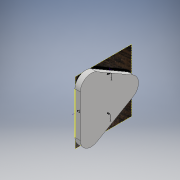
# Autodesk Inventor part: frontHub
Saved by Autodesk Inventor 2018 (Build 220112000, 112)
## iProperties
Created: 2019-07-29
Part Number: frontHub
Material: Generic
Document SubType Name: Modeling
Designer: Aditya Kendre
Density: 1 g/cm^3
Appearance: Default
Author: Aditya Kendre
Autodesk Inventor part; units mm, degrees
ref_plane "YZ Plane" through (0, 0, 0) normal (1, 0, 0) x (0, 1, 0)
ref_plane "XZ Plane" through (0, 0, 0) normal (0, 1, 0) x (-1, 0, 0)
ref_plane "XY Plane" through (0, 0, 0) normal (0, 0, 1) x (1, 0, 0)
sketch "Sketch1" plane through (0, 0, 0) normal (1, 0, 0) x (0, 1, 0)
  line L0 (0, 0) -> (12.7, 0) construction
  line L1 (12.7, 0) -> (-6.35, -10.9985)
  line L2 (-6.35, -10.9985) -> (-6.35, 10.9985)
  line L3 (-6.35, 10.9985) -> (12.7, 0)
  dimension "d0" = 12.7
  constraints: 8 end point, 1 coincident, 1 horizontal, 7 other
  measures "d0" distance of L0.start L0.end
extrude "Extrusion1" add sketch "Sketch1" along normal blind 1.5
fillet "Fillet1" radius 3 3 edges at (0.75, 12.7, 0) (0.75, -6.35, 10.9985) (0.75, -6.35, -10.9985)
sketch "Sketch2" plane through (0, 0, 0) normal (-1, 0, 0) x (0, 0, 1)
  line L0 (2.5981, 8.2) -> (8.4004, -1.85) construction
  line L1 (-8.4004, -1.85) -> (-2.5981, 8.2) construction
  line L2 (5.8024, -6.35) -> (-5.8024, -6.35) construction
  point P0 (0, 0)
  point P1 (5.4993, 3.175)
  point P2 (-5.4993, 3.175)
  point P3 (0, -6.35)
  constraints: 3 midpoint
sketch "Sketch3" plane through (0, 0, 0) normal (-1, 0, 0) x (0, 0, 1)
  line L0 (-8.571, 9.3033) -> (8.6339, 9.3033) construction
  line L1 (8.6339, 9.3033) -> (8.6339, -6.2748) construction
  line L2 (8.6339, -6.2748) -> (-8.571, -6.2748) construction
  line L3 (-8.571, -6.2748) -> (-8.571, 9.3033) construction
  line L4 (-5.8024, -6.35) -> (5.8024, -6.35) projected
  point P0 (0, 0)
  constraints: 1 parallel, 2 other
sketch "Sketch4" plane through (0, 0, 0) normal (-1, 0, 0) x (0, 0, 1)
  circle A0 centre (0, -5.358) radius 0.5
  circle A1 centre (-4.6765, 2.8681) radius 0.5
  circle A2 centre (4.7748, 2.8681) radius 0.5
  point P0 (0, 0)
  dimension "d126" = 1
  dimension "d127" = 1
  dimension "d128" = 1
  constraints: 3 centre point
  measures "d126" diameter of A0
  measures "d127" diameter of A1
  measures "d128" diameter of A2
body "Solid1"
